1.3mm_bottom (Autodesk Fusion 360 design; units mm, degrees)
Autodesk Fusion 360 part; units mm, degrees
note: some values were not read from the file. Set by a fixed rule: which sketch regions a step uses.
sketch "Sketch1" plane through (0, 0, 0) normal (0, 1, 0) x (1, 0, 0)
  line L0 (0, 0) -> (-0.5, 0)
  line L1 (-0.5, 0) -> (-0.5, -0.5895)
  line L2 (-0.5, -0.5895) -> (-0.049, -0.5895)
  line L3 (0, 0) -> (1.5, 0)
  line L4 (0, -0.46) -> (0, 0)
  line L5 (1.3, -0.46) -> (1.5, -0.375)
  line L6 (1.5, -0.375) -> (1.5, 0)
  line L7 (0, -0.46) -> (0.55, -0.46)
  line L8 (0.55, -0.46) -> (0.55, -0.41)
  line L9 (0.55, -0.41) -> (0.7, -0.41)
  line L10 (0.7, -0.41) -> (0.7, -0.46)
  line L11 (0.7, -0.46) -> (1.3, -0.46)
  line L12 (0, -0.46) -> (-0.05, -0.46)
  line L13 (-0.05, -0.46) -> (-0.0176, -0.5438)
  line L14 (-0.049, -0.5895) -> (-0.0176, -0.5438)
  line L15 (-0.049, -0.5895) -> (0, -0.5895) construction
  line L16 (-0.0176, -0.5438) -> (0, -0.5895) construction
  point P0 (0, -0.5895)
  dimension "d1" = 0.5
  dimension "d2" = 0.5895
  dimension "d6" = 0.375
  dimension "d7" = 0.2
  dimension "d8" = 2
  dimension "d11" = 0.55
  dimension "d12" = 0.15
  dimension "d13" = 0.46
  dimension "d14" = 0.05
  dimension "d21" = 0.05
  dimension "d24" = 0.049
  dimension "d25" = 0.049
  constraint horizontal L0
  constraint vertical L1
  constraint horizontal L2
  constraint coincident L0.start L3.start
  constraint horizontal L3
  constraint vertical L4
  constraint perpendicular L3 L6
  constraint perpendicular L7 L8
  constraint perpendicular L8 L9
  constraint perpendicular L9 L10
  constraint perpendicular L10 L11
  constraint collinear L7 L11
  constraint perpendicular L4 L12
  constraint vertical L0.start L15.end
  constraint coincident P0 L2
  constraint coincident P0 L13
  constraint coincident P0 L15.end
  constraint parallel L2 L15
  constraint parallel L13 L16
  measures "d1" distance of L1.end P0
  measures "d2" distance of L0.end L1.end
  measures "d6" distance of L3.end L5.end
  measures "d7" distance of L5.start L6
  measures "d8" distance of L1 L6
  measures "d11" distance of L4.start L7.end
  measures "d12" distance of L8.end L9.end
  measures "d13" distance of L3 L7
  measures "d14" distance of L9.end L10.end
  measures "d21" distance of L4.start L12.end
  measures "d24" distance of P0 L2.end
  measures "d25" distance of P0 L13.end
revolve "Revolve1" add sketch "Sketch1" angle 360 about axis through (0, 0, 0) along (1, 0, 0)
move_body "Move1" bodies 1 to x (0, 0, 1) y (0, 1, 0) z (-1, 0, 0) at (0, 0, 0)
equation "d2 = ( 1.179 / 2 ) * 1 mm"
equation "d13 = var / 2"
equation "var = 0.920 mm"
equation "d25 = d24"
